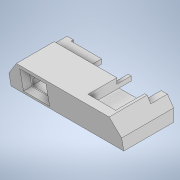
# Autodesk Inventor part: eonPCBcarrier
Saved by Autodesk Inventor 2020 (Build 240168000, 168)
## iProperties
Created: 2021-06-01
Part Number: eonPCBcarrier
Material: Generic
Document SubType Name: Modeling
Designer: dkiiv
Density: 1 g/cm^3
Appearance: Default
Author: dkiiv
Autodesk Inventor part; units mm, degrees
ref_plane "YZ Plane" through (0, 0, 0) normal (1, 0, 0) x (0, 1, 0)
ref_plane "XZ Plane" through (0, 0, 0) normal (0, 1, 0) x (-1, 0, 0)
sketch "Sketch1" plane through (0, 0, 0) normal (0, 0, 1) x (1, 0, 0)
  line L0 (0, 0) -> (51, 0)
  line L1 (51, 0) -> (51, 5.739)
  line L2 (51, 5.739) -> (0, 5.739) construction
  line L3 (0, 5.739) -> (0, 0)
  line L4 (4.5, 5.739) -> (46.5, 5.739)
  line L5 (46.5, 5.739) -> (46.5, 12.266) construction
  line L6 (46.5, 12.266) -> (4.5, 12.266)
  line L7 (4.5, 12.266) -> (4.5, 5.739) construction
  line L8 (4.5, 12.266) -> (0, 5.739)
  line L9 (46.5, 12.266) -> (51, 5.739)
  dimension "d0" = 51
  dimension "d1" = 5.739
  dimension "d2" = 42
  dimension "d3" = 4.5
  dimension "d4" = 12.266
  constraints: 20 end point, 4 parallel, 2 horizontal, 2 perpendicular, 1 point on line
  measures "d0" distance of L0.start L0.end
  measures "d1" distance of L2.end L0.start
  measures "d2" distance of L5.end L6.end
  measures "d3" distance between parallel lines of L3 L7
  measures "d4" distance between parallel lines of L0 L6
extrude "Extrusion1" add sketch "Sketch1" along normal blind 22.455
sketch "Sketch2" plane through (51, 0, 0) normal (1, 0, 0) x (0, 0, -1)
  line L0 (-22.455, 12.266) -> (-22.455, 5.739) projected
  line L1 (-22.455, 12.266) -> (-24.603, 12.266)
  line L2 (-22.455, 5.739) -> (-22.455, 0) projected
  line L3 (-24.603, 12.266) -> (-22.455, 0)
  line L4 (-22.455, 0) -> (-22.455, 12.266)
  point P0 (0, 0)
  dimension "d7" = 2.148
  constraints: 6 end point, 1 collinear, 1 horizontal
  measures "d7" distance of L0.start L1.end
extrude "Extrusion2" add sketch "Sketch2" against normal up to surface (51 mm away)
sketch "Sketch3" plane through (0, 0, 0) normal (0, 0, -1) x (-1, 0, 0)
  line L0 (-51, 5.739) -> (-46.5, 12.266) projected
  line L1 (-46.5, 12.266) -> (-51, 5.739)
  line L2 (-51, 5.739) -> (-60.9571, 11.6755)
  line L3 (-60.9571, 11.6755) -> (-47.5167, 21.4504)
  line L4 (-47.5167, 21.4504) -> (-46.5, 12.266)
  line L5 (-4.5, 12.266) -> (0, 12.266) projected
  line L6 (-46.5, 12.266) -> (-4.5, 12.266)
  line L7 (-4.5, 12.266) -> (0, 5.739) projected
  line L8 (-4.5, 12.266) -> (0, 5.739)
  line L9 (0, 5.739) -> (11.7434, 10.0464)
  line L10 (11.7434, 10.0464) -> (6.509, 19.8561)
  line L11 (6.509, 19.8561) -> (-3.5865, 15.5171)
  line L12 (-3.5865, 15.5171) -> (-4.5, 12.266)
  point P0 (0, 0)
  constraints: 20 end point, 3 collinear
extrude "Extrusion3" cut sketch "Sketch3" against normal up to surface surface through (51, 0, 22.455) normal (0, -0.1725, 0.985)
sketch "Sketch4" plane through (4.5, 12.266, 0) normal (0, 1, 0) x (1, 0, 0)
  line L0 (1.5, -1.193) -> (40.5, -1.193)
  line L1 (40.5, -1.193) -> (40.5, -20.193)
  line L2 (40.5, -20.193) -> (1.5, -20.193)
  line L3 (1.5, -20.193) -> (1.5, -1.193)
  line L4 (-4.5, 0) -> (-4.5, -23.46) projected
  line L5 (46.5, 0) -> (46.5, -23.46) projected
  line L6 (42, 0) -> (0, 0) projected
  dimension "d12" = 39
  dimension "d13" = 6
  dimension "d14" = 51
  dimension "d15" = 1.193
  dimension "d16" = 19
  constraints: 8 end point, 2 parallel, 1 horizontal, 1 perpendicular
  measures "d12" distance of L0.start L0.end
  measures "d13" distance between parallel lines of L4 L3
  measures "d14" distance between parallel lines of L5 L4
  measures "d15" distance between parallel lines of L6 L0
  measures "d16" distance of L2.end L0.start
extrude "Extrusion4" cut sketch "Sketch4" against normal blind 11.1
sketch "Sketch5" plane through (6, 12.266, 1.193) normal (0, 0, 1) x (1, 0, 0)
  line L0 (8.3, -6.1) -> (13.3, -6.1)
  line L1 (13.3, -6.1) -> (13.3, -3.6)
  line L2 (13.3, -3.6) -> (8.3, -3.6)
  line L3 (8.3, -3.6) -> (8.3, -6.1)
  line L4 (25.7, -6.1) -> (30.7, -6.1)
  line L5 (30.7, -6.1) -> (30.7, -3.6)
  line L6 (30.7, -3.6) -> (25.7, -3.6)
  line L7 (25.7, -3.6) -> (25.7, -6.1)
  line L8 (0, -11.1) -> (39, -11.1) projected
  line L9 (15.3, -4.0951) -> (23.7, -4.0951) construction
  line L10 (23.7, -4.0951) -> (23.7, -9.0951) construction
  line L11 (23.7, -9.0951) -> (15.3, -9.0951) construction
  line L12 (15.3, -9.0951) -> (15.3, -4.0951) construction
  line L13 (0, 0) -> (0, -11.1) projected
  line L14 (39, 0) -> (39, -11.1) projected
  point P0 (-6, -12.266)
  dimension "d19" = 5
  dimension "d20" = 5
  dimension "d23" = 2.5
  dimension "d24" = 5
  dimension "d25" = 0
  dimension "d26" = 5
  dimension "d27" = 8.4
  dimension "d28" = 5
  dimension "d29" = 15.3
  dimension "d30" = 15.3
  dimension "d31" = 2
  dimension "d32" = 2
  constraints: 24 end point, 6 parallel, 3 horizontal, 3 perpendicular
  measures "d19" distance of L0.start L0.end
  measures "d20" distance of L4.start L4.end
  measures "d23" distance of L6.end L4.start
  measures "d24" distance between parallel lines of L8 L4
  measures "d25" distance between parallel lines of L6 L2
  measures "d26" distance between parallel lines of L8 L0
  measures "d27" distance of L10.end L11.end
  measures "d28" distance of L9.end L10.end
  measures "d29" distance between parallel lines of L13 L12
  measures "d30" distance between parallel lines of L14 L10
  measures "d31" distance between parallel lines of L12 L1
  measures "d32" distance between parallel lines of L10 L7
extrude "Extrusion5" add sketch "Sketch5" along normal blind 6
sketch "Sketch6" plane through (4.5, 1.166, 0) normal (0, 1, 0) x (1, 0, 0)
  line L0 (10.75, -17.0266) -> (31.25, -17.0266)
  line L1 (31.25, -17.0266) -> (31.25, -19.2766)
  line L2 (31.25, -19.2766) -> (10.75, -19.2766)
  line L3 (10.75, -19.2766) -> (10.75, -17.0266)
  line L4 (1.5, -20.193) -> (1.5, -1.193) projected
  point P0 (-4.5, 0)
  dimension "d35" = 2.25
  dimension "d36" = 20.5
  dimension "d37" = 9.25
  constraints: 8 end point, 2 parallel, 1 horizontal, 1 perpendicular
  measures "d35" distance of L0.end L1.end
  measures "d36" distance of L0.start L0.end
  measures "d37" distance between parallel lines of L4 L3
extrude "Extrusion6" add sketch "Sketch6" along normal blind 1
sketch "Sketch7" plane through (45, 12.266, 20.193) normal (0, 0, -1) x (-1, 0, 0)
  line L0 (37, -7.5) -> (29.5, -7.5)
  line L1 (29.5, -7.5) -> (29.5, -3.8)
  line L2 (29.5, -3.8) -> (37, -3.8)
  line L3 (37, -3.8) -> (37, -7.5)
  line L4 (0, -11.1) -> (39, -11.1) projected
  line L5 (39, 0) -> (39, -11.1) projected
  line L6 (29.75, -10.1) -> (9.25, -10.1) projected
  point P0 (45, -12.266)
  dimension "d40" = 7.5
  dimension "d41" = 3.7
  dimension "d43" = 2
  dimension "d106" = 2.6
  constraints: 8 end point, 2 parallel, 1 horizontal, 1 perpendicular
  measures "d40" distance of L1.end L2.end
  measures "d41" distance of L0.end L1.end
  measures "d43" distance between parallel lines of L5 L3
  measures "d106" distance between parallel lines of L0 L6
extrude "Extrusion7" cut sketch "Sketch7" against normal blind 8.25
sketch "Sketch9" plane through (4.5, 1.166, 0) normal (0, 1, 0) x (1, 0, 0)
  line L0 (9.8, -7.193) -> (14.8, -7.193) projected
  circle A0 centre (9.8, -7.193) radius 0.5
  circle A1 centre (14.8, -7.193) radius 0.5
  circle A2 centre (27.2, -7.193) radius 0.5
  line L1 (27.2, -7.193) -> (32.2, -7.193) projected
  circle A3 centre (32.2, -7.193) radius 0.5
  point P0 (-4.5, 0)
  dimension "d51" = 1
  dimension "d52" = 1
  dimension "d53" = 1
  dimension "d54" = 1
  constraints: 4 centre point, 1 coincident
  measures "d51" diameter of A0
  measures "d52" diameter of A1
  measures "d53" diameter of A2
  measures "d54" diameter of A3
extrude "Extrusion9" add sketch "Sketch9" along normal blind 1
sketch "Sketch10" plane through (14.3, 2.166, 7.193) normal (0, 1, 0) x (1, 0, 0)
  line L0 (0, 0) -> (5, 0) projected
  circle A0 centre (0, 0) radius 1
  line L1 (5, 6) -> (5, 0) projected
  circle A1 centre (5, 0) radius 1
  circle A2 centre (17.4, 0) radius 0.5 projected
  circle A3 centre (17.4, 0) radius 1
  line L2 (17.4, 0) -> (22.4, 0) projected
  circle A4 centre (22.4, 0) radius 1
  point P0 (-14.3, 7.193)
  dimension "d57" = 2
  dimension "d58" = 2
  dimension "d59" = 2
  dimension "d60" = 2
  constraints: 4 centre point, 2 coincident
  measures "d57" diameter of A0
  measures "d58" diameter of A1
  measures "d59" diameter of A3
  measures "d60" diameter of A4
extrude "Extrusion10" add sketch "Sketch10" along normal blind 3 contours A1 L1 L0 | L0 L1 A1 | A0 | A2 | A3 | A4
sketch "Sketch11" plane through (14.3, 5.166, 7.193) normal (0, 1, 0) x (1, 0, 0)
  circle A0 centre (0, 0) radius 0.5 projected
  circle A1 centre (0, 0) radius 0.5
  circle A2 centre (5, 0) radius 0.5 projected
  circle A3 centre (5, 0) radius 0.5
  circle A4 centre (17.4, 0) radius 0.5 projected
  circle A5 centre (17.4, 0) radius 0.5
  circle A6 centre (22.4, 0) radius 0.5 projected
  circle A7 centre (22.4, 0) radius 0.5
  point P0 (-14.3, 7.193)
  constraints: 4 centre point, 4 coincident
extrude "Extrusion11" add sketch "Sketch11" along normal blind 1
ref_plane "Work Plane1" through (4.65, 12.116, 0) normal (0, 1, 0) x (1, 0, 0)
sketch "Sketch13" plane through (4.65, 12.116, 0) normal (0, 1, 0) x (1, 0, 0)
  line L0 (40.35, -20.193) -> (1.35, -20.193) projected
  line L1 (1.35, -20.193) -> (40.35, -20.193)
  line L2 (40.35, -20.193) -> (40.35, -20.343)
  line L3 (40.35, -20.343) -> (1.35, -20.343)
  line L4 (40.35, -20.343) -> (40.5, -20.343)
  line L5 (40.5, -20.343) -> (40.5, -1.193)
  line L6 (40.5, -1.193) -> (40.35, -1.193)
  line L7 (40.35, -1.193) -> (40.35, -20.343)
  line L8 (40.5, -1.193) -> (1.35, -1.193)
  line L9 (1.35, -1.193) -> (1.35, -1.043)
  line L10 (1.35, -1.043) -> (40.5, -1.043)
  line L11 (40.5, -1.043) -> (40.5, -1.193)
  line L12 (1.35, -1.043) -> (1.2, -1.043)
  line L13 (1.2, -1.043) -> (1.2, -20.343)
  line L14 (1.2, -20.343) -> (1.35, -20.343)
  line L15 (1.35, -20.193) -> (1.35, -1.043)
  point P0 (-4.65, 0)
  point P1 (1.35, -20.193)
  point P2 (1.35, -1.193)
  dimension "d77" = 0.15
  dimension "d78" = 0.15
  dimension "d79" = 0.15
  dimension "d80" = 0.15
  constraints: 30 end point, 7 parallel, 4 horizontal, 4 perpendicular, 2 point on line
  measures "d77" distance of L1.end L2.end
  measures "d78" distance of L6.end L5.end
  measures "d79" distance of L8.end L9.end
  measures "d80" distance of L14.end L13.end
extrude "Extrusion13" cut sketch "Sketch13" along normal blind 10.95 and the other way blind 10.95 contours L2 L3 L14 L13 L12 L9 L15 L0 | L7 L6 L5 L4 L2 | L8 L9 L10 L11 L6
sketch "Sketch14" plane through (14.3, 8.666, 7.193) normal (0, 1, 0) x (1, 0, 0)
  line L0 (0, 6) -> (5, 6) projected
  line L1 (0, 6) -> (5, 6)
  line L2 (5, 6) -> (5, 6.15)
  line L3 (5, 6.15) -> (0, 6.15)
  line L4 (0, 6.15) -> (0, 6)
  line L5 (17.4, 6) -> (17.4, 0) projected
  line L6 (17.4, 6) -> (22.4, 6)
  line L7 (22.4, 6) -> (22.4, 6.15)
  line L8 (22.4, 6.15) -> (17.4, 6.15)
  line L9 (17.4, 6.15) -> (17.4, 6)
  point P0 (-14.3, 7.193)
  dimension "d83" = 5
  dimension "d84" = 0.15
  dimension "d85" = 5
  dimension "d86" = 0.15
  constraints: 16 end point, 4 parallel, 2 horizontal, 2 perpendicular
  measures "d83" distance of L3.end L2.end
  measures "d84" distance of L2.end L1.end
  measures "d85" distance of L8.end L7.end
  measures "d86" distance of L7.end L6.end
extrude "Extrusion14" add sketch "Sketch14" against normal up to surface (2.5 mm away)
sketch "Sketch16" plane through (4.5, 12.266, 24.603) normal (0, 1, 0) x (1, 0, 0)
  line L0 (1.35, 23.56) -> (40.65, 23.56) projected
  line L1 (1.35, 23.56) -> (1.2, 23.56)
  line L2 (1.2, 23.56) -> (1.2, 4.11)
  line L3 (1.2, 4.11) -> (1.35, 4.11)
  line L4 (1.35, 4.11) -> (1.35, 23.56)
  line L5 (40.65, 4.26) -> (1.35, 4.26) projected
  line L6 (40.65, 4.26) -> (1.35, 4.26) projected
  line L7 (1.35, 4.11) -> (40.65, 4.11)
  line L8 (40.65, 4.11) -> (40.65, 4.26)
  line L9 (40.65, 4.26) -> (1.35, 4.26)
  line L10 (1.35, 4.26) -> (1.35, 4.11)
  line L11 (40.65, 4.11) -> (40.8, 4.11)
  line L12 (40.8, 4.11) -> (40.8, 23.56)
  line L13 (40.8, 23.56) -> (40.65, 23.56)
  line L14 (40.65, 23.56) -> (40.65, 4.11)
  point P0 (-4.5, 24.603)
  point P1 (14.8, 23.56)
  point P2 (40.65, 4.26)
  dimension "d96" = 0.15
  dimension "d97" = 0.15
  dimension "d98" = 0.15
  constraints: 24 end point, 6 parallel, 3 horizontal, 3 perpendicular
  measures "d96" distance of L3.end L2.end
  measures "d97" distance between parallel lines of L5 L3
  measures "d98" distance of L0.end L12.end
extrude "Extrusion16" cut sketch "Sketch16" against normal up to surface (11.1 mm away) contours L4 L3 L2 L1 | L13 L12 L11 L8 L14 | L5 L8 L7 L4
sketch "Sketch17" plane through (14.3, 8.666, 7.193) normal (0, 1, 0) x (1, 0, 0)
  line L0 (31, 6.15) -> (-8.6, 6.15) projected
  line L1 (-3.1355, -2.3842) -> (26.7601, -2.3842)
  line L2 (26.7601, -2.3842) -> (26.7601, 6.15)
  line L3 (26.7601, 6.15) -> (-3.1355, 6.15)
  line L4 (-3.1355, 6.15) -> (-3.1355, -2.3842)
  point P0 (-14.3, 7.193)
  point P1 (-3.1355, 6.15)
  constraints: 8 end point, 2 parallel, 1 horizontal, 1 perpendicular, 1 point on line
extrude "Extrusion17" cut sketch "Sketch17" against normal up to surface (7.5 mm away)
sketch "Sketch18" plane through (45.3, 12.266, 20.493) normal (0, 0, -1) x (-1, 0, 0)
  line L0 (37.3, -3.8) -> (29.8, -3.8) projected
  line L1 (29.8, -7.5) -> (37.3, -7.5) projected
  line L2 (29.8, -3.8) -> (37.3, -3.8)
  line L3 (37.3, -3.8) -> (37.3, -7.5)
  line L4 (37.3, -7.5) -> (29.8, -7.5)
  line L5 (29.8, -6.6) -> (29.8, -3.8)
  line L6 (0, -10.1) -> (39.6, -10.1)
  line L7 (39.6, -10.1) -> (39.6, -6.6)
  line L8 (0, -6.6) -> (0, -10.1)
  line L9 (39.6, -11.1) -> (0, -11.1) projected
  line L10 (0, 0) -> (0, -11.1) projected
  line L11 (39.6, 0) -> (39.6, -11.1) projected
  line L12 (12.4908, -6.6) -> (0, -6.6)
  line L13 (0, -6.6) -> (0, 1.6477)
  line L14 (0, 1.6477) -> (12.4908, 1.6477)
  line L15 (12.4908, 1.6477) -> (12.4908, -6.6)
  line L16 (39.6, -6.6) -> (37.3, -6.6)
  line L17 (29.8, -6.6) -> (0, -6.6)
  point P0 (45.3, -12.266)
  point P1 (37.3, -3.8)
  dimension "d107" = 1
  dimension "d108" = 0
  dimension "d109" = 0
  dimension "d110" = 3.5
  constraints: 26 end point, 7 parallel, 3 horizontal, 3 perpendicular, 3 point on line
  measures "d107" distance between parallel lines of L9 L6
  measures "d108" distance between parallel lines of L10 L8
  measures "d109" distance between parallel lines of L11 L7
  measures "d110" distance of L8.start L6.start
extrude "Extrusion18" cut sketch "Sketch18" along normal up to surface (20.493 mm away) contours L3 L16 L7 L6 L8 L12 L17 L5 L0 | L12 L10 L13 L14 L15
sketch "Sketch19" plane through (5.7, 12.266, 1.043) normal (0, 0, 1) x (1, 0, 0)
  line L0 (0, 0) -> (0, -6.6) projected
  line L1 (0, 0) -> (0, -6.6)
  line L2 (0, -6.6) -> (2.3, -6.6) projected
  line L3 (0, -6.6) -> (2.3, -6.6)
  line L4 (2.3, -3.8) -> (2.3, -6.6) projected
  line L5 (2.3, -6.6) -> (2.3, -3.8)
  line L6 (9.8, -6.6) -> (9.8, -3.8) projected
  line L7 (2.3, -3.8) -> (9.8, -3.8)
  line L8 (9.8, -6.6) -> (27.1092, -6.6) projected
  line L9 (9.8, -3.8) -> (9.8, -6.6)
  line L10 (9.8, -6.6) -> (27.1092, -6.6)
  line L11 (27.1092, 0) -> (27.1092, -6.6) projected
  line L12 (27.1092, -6.6) -> (27.1092, 0)
  line L13 (0, 0) -> (27.1092, 0) projected
  line L14 (27.1092, 0) -> (0, 0)
  point P0 (-5.7, -12.266)
  constraints: 16 end point, 5 perpendicular, 2 collinear, 1 vertical
extrude "Extrusion19" add sketch "Sketch19" along normal up to surface (19.45 mm away)
chamfer "Chamfer5" distance 1 angle 45 1 edges at (25.5, 1.166, 19.2766)
sketch "Sketch20" plane through (4.5, 12.266, 24.603) normal (0, 1, 0) x (1, 0, 0)
  line L0 (27, 23.56) -> (15, 23.56)
  line L1 (15, 23.56) -> (15, 18.06)
  line L2 (15, 18.06) -> (27, 18.06)
  line L3 (27, 18.06) -> (27, 23.56)
  line L4 (42, 24.603) -> (42, 0) projected
  line L5 (40.8, 23.56) -> (1.2, 23.56) projected
  line L6 (40.8, 4.11) -> (40.8, 23.56) projected
  line L7 (28.3092, 24.603) -> (0, 24.603) projected
  line L8 (40.8, 23.56) -> (0, 23.56)
  line L9 (0, 23.56) -> (0, 24.603)
  line L10 (0, 24.603) -> (40.8, 24.603)
  line L11 (40.8, 24.603) -> (40.8, 23.56)
  line L12 (1.2, 23.56) -> (1.2, 24.603) projected
  line L13 (1.2, 23.56) -> (1.2, 24.603)
  point P0 (-4.5, 24.603)
  point P1 (28.3092, 24.603)
  dimension "d118" = 12
  dimension "d119" = 5.5
  dimension "d120" = 15
  dimension "d121" = 0
  constraints: 18 end point, 5 equal length, 2 horizontal, 2 perpendicular
  measures "d118" distance of L2.end L1.end
  measures "d119" distance of L1.end L0.end
  measures "d120" distance between parallel lines of L4 L3
  measures "d121" distance between parallel lines of L5 L0
extrude "Extrusion20" cut sketch "Sketch20" against normal up to surface (11.1 mm away) contours L3 L2 L1 L0 | L0 L5 L12 L7 L10 L11
sketch "Sketch21" plane through (19.5, 12.266, 1.043) normal (0, 0, -1) x (-1, 0, 0)
  line L0 (11.65, -3.65) -> (3.85, -3.65)
  line L1 (3.85, -3.65) -> (3.85, -7.65)
  line L2 (3.85, -7.65) -> (11.65, -7.65)
  line L3 (11.65, -7.65) -> (11.65, -3.65)
  line L4 (4, -7.5) -> (11.5, -7.5) projected
  line L5 (11.5, -6.6) -> (11.5, -3.8) projected
  line L6 (11.5, -3.8) -> (4, -3.8) projected
  line L7 (4, -3.8) -> (4, -6.6) projected
  point P0 (19.5, -12.266)
  dimension "d127" = 0.15
  dimension "d128" = 0.15
  dimension "d129" = 0.15
  dimension "d130" = 0.15
  constraints: 8 end point, 2 parallel, 1 horizontal, 1 perpendicular
  measures "d127" distance between parallel lines of L4 L2
  measures "d128" distance between parallel lines of L5 L3
  measures "d129" distance between parallel lines of L6 L0
  measures "d130" distance between parallel lines of L1 L7
extrude "Extrusion21" cut sketch "Sketch21" against normal blind 31.75
sketch "Sketch22" plane through (0, 0, 0) normal (0, 0, -1) x (-1, 0, 0)
  line L0 (0, 0) -> (-51, 0) projected
  line L1 (-48.0686, 0.075) -> (-48.0686, 5.664)
  line L2 (-48.0686, 5.664) -> (-50.925, 5.664)
  line L3 (-50.925, 5.664) -> (-50.925, 0)
  line L4 (-51, 0) -> (-51, 5.739) projected
  line L5 (-46.425, 12.191) -> (-4.575, 12.191)
  line L6 (-4.575, 12.191) -> (-4.575, 10.7889)
  line L7 (-4.575, 10.7889) -> (-46.425, 10.7889)
  line L8 (-46.425, 10.7889) -> (-46.425, 12.191)
  line L9 (-46.5, 12.266) -> (-45.3, 12.266) projected
  line L10 (-46.425, 12.191) -> (-50.925, 5.664)
  line L11 (-4.5, 12.266) -> (0, 5.739) projected
  line L12 (-4.5, 12.266) -> (-4.5, 12.191)
  line L13 (-0.075, 5.664) -> (-3.316, 5.664)
  line L14 (-3.316, 5.664) -> (-3.316, 0.075)
  line L15 (-3.316, 0.075) -> (-0.075, 0.075)
  line L16 (-0.075, 0.075) -> (-0.075, 5.664)
  line L17 (0, 5.739) -> (0, 0) projected
  line L18 (-2.5152, 0.075) -> (-50.925, 0.075)
  line L19 (-4.575, 12.191) -> (-0.075, 5.664)
  line L20 (-56.1384, 19.3089) -> (5.3799, 19.3089)
  line L21 (5.3799, 19.3089) -> (5.3799, -4.8972)
  line L22 (5.3799, -4.8972) -> (-56.1384, -4.8972)
  line L23 (-56.1384, -4.8972) -> (-56.1384, 19.3089)
  point P0 (-3.316, 0.075)
  dimension "d133" = 0.075
  dimension "d134" = 0.075
  dimension "d135" = 0.075
  dimension "d136" = 0.075
  dimension "d137" = 0.075
  dimension "d138" = 0.075
  dimension "d139" = 0.075
  dimension "d140" = 0.075
  constraints: 38 end point, 7 parallel, 6 point on line, 3 horizontal, 3 perpendicular, 1 vertical
  measures "d133" distance between parallel lines of L4 L3
  measures "d134" distance from line of L4.end L2
  measures "d135" distance between parallel lines of L9 L5
  measures "d136" distance from line of L9.start L8
  measures "d137" distance between parallel lines of L12 L6
  measures "d138" distance between parallel lines of L17 L16
  measures "d139" distance between parallel lines of L0 L15
  measures "d140" distance from line of L11.end L13
extrude "Extrusion22" cut sketch "Sketch22" against normal blind 29
sketch "Sketch23" plane through (15.65, 8.616, 1.043) normal (0, 0, -1) x (-1, 0, 0)
  line L0 (0, -2.95) -> (0, 0) projected
  line L1 (0, 0) -> (7.8, 0)
  line L2 (7.8, 0) -> (7.8, -5.6)
  line L3 (7.8, -5.6) -> (0, -5.6)
  line L4 (0, -5.6) -> (0, 0)
  line L5 (7.8, -4) -> (0, -4) projected
  line L6 (0, -2.95) -> (-17.1592, -2.95) projected
  line L7 (-17.1592, -2.95) -> (-17.1592, 3.575) projected
  line L8 (0, -2.95) -> (-17.1592, -2.95)
  line L9 (-17.1592, -2.95) -> (-17.1592, -0.95)
  line L10 (-17.1592, -0.95) -> (0, -0.95)
  line L11 (0, -0.95) -> (0, -2.95)
  point P0 (15.65, -8.616)
  point P1 (0, -0.95)
  dimension "d143" = 1.6
  dimension "d144" = 2
  constraints: 16 end point, 4 parallel, 2 horizontal, 2 perpendicular, 1 point on line
  measures "d143" distance between parallel lines of L3 L5
  measures "d144" distance of L8.end L9.end
extrude "Extrusion23" cut sketch "Sketch23" against normal up to surface contours L0 L1 L2 L5 L4 | L5 L2 L3 L4 surface through (51, 0, 22.455) normal (0, -0.1725, 0.985)
extrude "Extrusion24" cut sketch "Sketch23" against normal up to surface (19.45 mm away) contours L6 L7 L10 L0
chamfer "Chamfer7" distance 2 angle 45 4 edges at (11.75, 8.616, 23.9638) (7.85, 5.816, 23.4735) (15.65, 5.816, 23.4735) (11.75, 3.016, 22.9832)
sketch "Sketch24" plane through (0, 0, 0) normal (0, 0, -1) x (-1, 0, 0)
  line L0 (-51.2021, 14.8719) -> (1.5276, 14.8719)
  line L1 (1.5276, 14.8719) -> (1.5276, 9.691)
  line L2 (1.5276, 9.691) -> (-51.2021, 9.691)
  line L3 (-51.2021, 9.691) -> (-51.2021, 14.8719)
  line L4 (-45.3, 12.191) -> (-46.425, 12.191) projected
  point P0 (0, 0)
  dimension "d152" = 2.5
  constraints: 8 end point, 2 parallel, 1 horizontal, 1 perpendicular
  measures "d152" distance between parallel lines of L4 L2
extrude "Extrusion25" cut sketch "Sketch24" against normal blind 7.5
body "Solid1"
